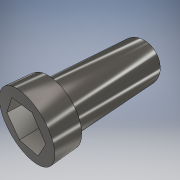
# Autodesk Inventor part: nut
Saved by Autodesk Inventor 2018 (Build 220112000, 112)
## iProperties
Created: 2021-01-31
Part Number: nut
Material: Všeobecné
Document SubType Name: Modeling
Designer: Jozko Mrkvicka
Density: 1 g/cm^3
Appearance: Ocel – leštěná
Author: Jozko Mrkvicka
Autodesk Inventor part; units mm, degrees
ref_plane "YZ Plane" through (0, 0, 0) normal (1, 0, 0) x (0, 1, 0)
ref_plane "XZ Plane" through (0, 0, 0) normal (0, 1, 0) x (-1, 0, 0)
ref_plane "XY Plane" through (0, 0, 0) normal (0, 0, 1) x (1, 0, 0)
sketch "Náčrt1" plane through (0, 0, 0) normal (0, 1, 0) x (-1, 0, 0)
  circle A0 centre (0, 0) radius 4
  dimension "nutOuterDia" = 8
  constraints: 1 centre point, 1 coincident
  measures "nutOuterDia" diameter of A0
extrude "Vysunutí2" add sketch "Náčrt1" along normal blind 16
sketch "Náčrt3" plane through (0, 0, 0) normal (0, -1, 0) x (1, 0, 0)
  circle A0 centre (0, 0) radius 4 projected
  line L0 (-2.8868, 0) -> (-1.4434, 2.5)
  line L1 (-1.4434, 2.5) -> (1.4434, 2.5)
  line L2 (1.4434, 2.5) -> (2.8868, 0)
  line L3 (2.8868, 0) -> (1.4434, -2.5)
  line L4 (1.4434, -2.5) -> (-1.4434, -2.5)
  line L5 (-1.4434, -2.5) -> (-2.8868, 0)
  dimension "keyHoleSize" = 5
  constraints: 12 end point, 1 coincident, 13 other
  measures "keyHoleSize" distance between parallel lines of L3 L0
extrude "Vysunutí3" cut sketch "Náčrt3" against normal blind 3 contours L0 L1 L2 L3 L4 L5
sketch "Náčrt4" plane through (0, 16, 0) normal (0, 1, 0) x (1, 0, 0)
  circle A0 centre (0, 0) radius 4 projected
  circle A1 centre (0, 0) radius 3
  constraints: 1 centre point, 1 coincident
extrude "Vysunutí4" cut sketch "Náčrt4" against normal blind 13
sketch "Náčrt5" plane through (0, 16, 0) normal (0, 1, 0) x (1, 0, 0)
  circle A0 centre (0, 0) radius 3 projected
  circle A1 centre (0, 0) radius 2
  constraints: 1 centre point, 1 coincident
extrude "Vysunutí5" cut sketch "Náčrt5" against normal blind 10 contours A1
thread "Závit2" size "M4x0.7" class "6H" standard "ANSI Metric M Profile" full length
